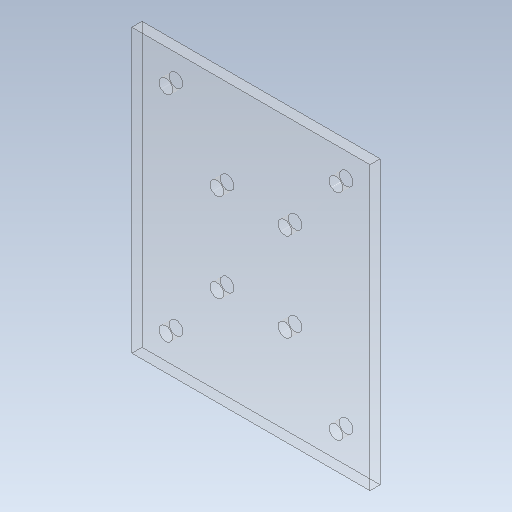
# Autodesk Inventor part: BaseC_8
Saved by Autodesk Inventor 2021.1 (Build 251245010, 245A)
## iProperties
Created: 2023-10-22
Part Number: BaseC_8
Material: PMMA Plastic
Document SubType Name: Modeling
Designer: M
Density: 1.188 g/cm^3
Appearance: Polycarbonate - Clear
Author: M
Autodesk Inventor part; units mm, degrees
ref_plane "YZ Plane" through (0, 0, 0) normal (1, 0, 0) x (0, 1, 0)
ref_plane "XZ Plane" through (0, 0, 0) normal (0, 1, 0) x (-1, 0, 0)
ref_plane "XY Plane" through (0, 0, 0) normal (0, 0, 1) x (1, 0, 0)
sketch "Sketch1" plane through (0, 0, 0) normal (0, 0, 1) x (1, 0, 0)
  line L0 (73, -75) -> (3, -75)
  line L1 (3, 8) -> (3, -75)
  line L2 (3, 8) -> (73, 8)
  line L3 (73, 8) -> (73, -75)
  circle A0 centre (13, -65) radius 2
  circle A1 centre (13, -2) radius 2
  circle A2 centre (63, -65) radius 2
  circle A3 centre (63, -2) radius 2
  circle A4 centre (28, -46.5) radius 2
  circle A5 centre (48, -46.5) radius 2
  line L4 (28, -46.5) -> (48, -46.5)
  circle A6 centre (28, -20.5) radius 2
  circle A7 centre (48, -20.5) radius 2
  line L5 (28, -20.5) -> (48, -20.5)
  point P0 (0, 0)
  dimension "d0" = 70
  dimension "d1" = 83
  dimension "d4" = 4
  dimension "d5" = 10
  dimension "d6" = 10
  dimension "d7" = 4
  dimension "d8" = 4
  dimension "d9" = 4
  dimension "d10" = 10
  dimension "d11" = 10
  dimension "d12" = 10
  dimension "d13" = 10
  dimension "d14" = 10
  dimension "d15" = 10
  dimension "d16" = 4
  dimension "d17" = 20
  dimension "d18" = 4
  dimension "d19" = 4
  dimension "d20" = 20
  dimension "d21" = 4
  dimension "d22" = 26
  dimension "d23" = 28.5
  dimension "d24" = 25
  constraints: 12 end point, 8 centre point, 2 horizontal, 1 vertical
  measures "d0" distance of L0.start L0.end
  measures "d1" distance of L1.start L0.end
  measures "d4" diameter of A0
  measures "d5" distance from line of A0.centre L1
  measures "d6" distance from line of L0 A0.centre
  measures "d7" diameter of A1
  measures "d8" diameter of A2
  measures "d9" diameter of A3
  measures "d10" distance from line of L1 A1.centre
  measures "d11" distance from line of L2 A1.centre
  measures "d12" distance from line of L0 A2.centre
  measures "d13" distance from line of L3 A2.centre
  measures "d14" distance from line of L3 A3.centre
  measures "d15" distance from line of L2 A3.centre
  measures "d16" diameter of A4
  measures "d17" distance of L4.start L4.end
  measures "d18" diameter of A5
  measures "d19" diameter of A6
  measures "d20" distance of L5.start L5.end
  measures "d21" diameter of A7
  measures "d22" distance of L5.start L4.start
  measures "d23" distance from line of L0 L4.start
  measures "d24" distance from line of L1 L4.start
extrude "Extrusion1" add sketch "Sketch1" along normal blind 3
equation "\"d10\" = d5"
equation "\"d11\" = d6"
equation "\"d13\" = d12"
equation "\"d14\" = d13"
equation "\"d15\" = d14"
equation "\"d18\" = d16"
equation "\"d21\" = d19"
equation "\"d23\" = -0.5 * d22 + 0.5 * d1"
equation "\"d24\" = -0.5 * d17 + 0.5 * d0"
body "Solid1"
